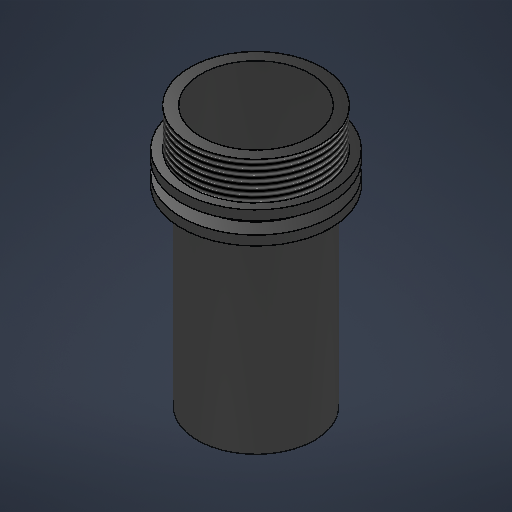
# Autodesk Inventor part: Plunger
Saved by Autodesk Inventor 2026 (Build 300175050, 175E)
## iProperties
Created: 2025-06-28
Part Number: Plunger
Material: ABS Plastic
Document SubType Name: Modeling
Designer: Joshua Eah
Density: 1.06 g/cm^3
Appearance: Glossy - Black
Author: Joshua Eah
Autodesk Inventor part; units mm, degrees
ref_plane "YZ Plane" through (0, 0, 0) normal (1, 0, 0) x (0, 1, 0)
ref_plane "XZ Plane" through (0, 0, 0) normal (0, 1, 0) x (-1, 0, 0)
ref_plane "XY Plane" through (0, 0, 0) normal (0, 0, 1) x (1, 0, 0)
sketch "Sketch1" plane through (0, 0, 0) normal (0, 1, 0) x (-1, 0, 0)
  circle A0 centre (0, 0) radius 7.75
  dimension "d0" = 15.5
  constraints: 1 centre point, 1 coincident
  measures "d0" diameter of A0
extrude "Extrusion1" add sketch "Sketch1" along normal blind 25.4
sketch "Sketch2" plane through (0, 25.4, 0) normal (0, 1, 0) x (1, 0, 0)
  circle A0 centre (0, 0) radius 7.75 projected
  circle A1 centre (0, 0) radius 9.875
  dimension "d3" = 19.75
  constraints: 1 centre point, 1 coincident
  measures "d3" diameter of A1
extrude "Extrusion2" add sketch "Sketch2" along normal blind 1.25 contours A0 | A1
sketch "Sketch3" plane through (0, 26.65, 0) normal (0, 1, 0) x (1, 0, 0)
  circle A0 centre (0, 0) radius 9.875 projected
  circle A1 centre (0, 0) radius 7.75
  dimension "d6" = 15.5
  constraints: 1 centre point, 1 coincident
  measures "d6" diameter of A1
extrude "Extrusion3" add sketch "Sketch3" along normal blind 1.65 contours A1
sketch "Sketch4" plane through (0, 28.3, 0) normal (0, 1, 0) x (1, 0, 0)
  circle A0 centre (0, 0) radius 7.75 projected
  circle A1 centre (0, 0) radius 9.875
  dimension "d9" = 19.75
  constraints: 1 centre point, 1 coincident
  measures "d9" diameter of A1
extrude "Extrusion4" add sketch "Sketch4" along normal blind 1.25 contours A0 | A1
sketch "Sketch5" plane through (0, 29.55, 0) normal (0, 1, 0) x (1, 0, 0)
  circle A0 centre (0, 0) radius 9.875 projected
  circle A1 centre (0, 0) radius 8.75
  dimension "d12" = 17.5
  constraints: 1 centre point, 1 coincident
  measures "d12" diameter of A1
extrude "Extrusion5" add sketch "Sketch5" along normal blind 5 contours A1
thread "Thread1" size "M18x0.75" class "6g" standard "ANSI Metric M Profile" full length
hole "Hole1" at (0, 0, 0) direction (0, 1, 0) diameter 14.5 end through all
body "Solid1"
